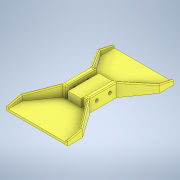
# Autodesk Inventor part: Base
Saved by Autodesk Inventor 2022.4 (Build 264492000, 492)
## iProperties
Created: 2024-03-21
Part Number: Base
Material: Generic
Document SubType Name: Modeling
Designer: t60147996
Density: 1 g/cm^3
Appearance: Smooth - Yellow
Author: t60147996
Autodesk Inventor part; units mm, degrees
ref_plane "YZ Plane" through (0, 0, 0) normal (1, 0, 0) x (0, 1, 0)
ref_plane "XZ Plane" through (0, 0, 0) normal (0, 1, 0) x (-1, 0, 0)
ref_plane "XY Plane" through (0, 0, 0) normal (0, 0, 1) x (1, 0, 0)
sketch "Sketch1" plane through (0, 0, 0) normal (0, 1, 0) x (-1, 0, 0)
  line L0 (88.9, 152.4) -> (-88.9, 152.4)
  line L1 (-88.9, 152.4) -> (-88.9, -152.4)
  line L2 (-88.9, -152.4) -> (88.9, -152.4)
  line L3 (88.9, -152.4) -> (88.9, 152.4)
  line L4 (88.9, 152.4) -> (-88.9, -152.4) construction
  line L5 (-88.9, 152.4) -> (88.9, -152.4) construction
  point P0 (0, 0)
  dimension "d2" = 177.8
  dimension "d3" = 304.8
  constraints: 12 end point, 2 midpoint, 2 parallel, 1 horizontal, 1 perpendicular
  measures "d2" distance of L2.end L1.end
  measures "d3" distance of L1.end L0.end
extrude "Extrusion1" add sketch "Sketch1" along normal blind 38.1
sketch "Sketch2" plane through (0, 38.1, 0) normal (0, 1, 0) x (1, 0, 0)
  line L0 (-88.9, -110.6499) -> (-38.1, -38.1)
  line L1 (-38.1, -38.1) -> (-38.1, 38.1)
  line L2 (-88.9, 152.4) -> (-88.9, -152.4) projected
  line L3 (-38.1, 38.1) -> (-88.9, 110.6499)
  line L4 (-88.9, -110.6499) -> (-88.9, 110.6499)
  point P0 (0, 0)
  point P1 (-38.1, 0)
  point P2 (-88.9, 0)
  point P3 (-88.9, 0)
  dimension "d8" = 50.8
  dimension "d9" = 35
  dimension "d10" = 35
  dimension "d11" = 114.3
  constraints: 8 end point, 3 midpoint, 1 coincident, 1 horizontal alignment, 1 parallel, 1 vertical
  measures "d8" distance between parallel lines of L4 L1
  measures "d9" angle of L4 L3
  measures "d10" angle of L4 L0
  measures "d11" vertical distance of L2.end L0.end
extrude "Extrusion2" cut sketch "Sketch2" against normal blind 38.1
mirror "Mirror1" about plane through (0, 0, 0) normal (1, 0, 0) of "Extrusion2"
sketch "Sketch3" plane through (-88.9, 0, -152.4) normal (-1, 0, 0) x (0, 0, 1)
  line L0 (41.7501, 38.1) -> (114.3, 38.1) projected
  line L1 (114.3, 38.1) -> (0, 12.7)
  line L2 (0, 0) -> (0, 38.1) projected
  line L3 (0, 38.1) -> (41.7501, 38.1) projected
  line L4 (0, 0) -> (41.7501, 0) projected
  point P0 (152.4, 0)
  constraints: 2 end point, 1 point on line
extrude "Extrusion3" cut sketch "Sketch3" against normal through all
mirror "Mirror2" about plane through (0, 0, 0) normal (0, 0, 1) of "Extrusion3"
sketch "Sketch4" plane through (0, 38.1, 0) normal (0, 1, 0) x (1, 0, 0)
  line L0 (88.9, 152.4) -> (88.9, 110.6499) projected
  line L1 (88.9, 110.6499) -> (38.1, 38.1) projected
  line L2 (38.1, 38.1) -> (-38.1, 38.1) projected
  line L3 (-38.1, 38.1) -> (-88.9, 110.6499) projected
  line L4 (-88.9, 110.6499) -> (-88.9, 152.4) projected
  line L5 (-82.55, 175.6071) -> (-82.55, 112.6521)
  line L6 (-82.55, 112.6521) -> (-34.7944, 44.45)
  line L7 (-34.7944, 44.45) -> (34.7944, 44.45)
  line L8 (34.7944, 44.45) -> (82.55, 112.6521)
  line L9 (82.55, 112.6521) -> (82.55, 175.6071)
  line L10 (82.55, 175.6071) -> (-82.55, 175.6071)
  line L11 (-88.9, 152.4) -> (-88.9, 110.6499) projected
  point P0 (0, 0)
  dimension "d18" = 6.35
  constraints: 12 end point, 1 perpendicular, 4 other
  measures "d18" distance between parallel lines of L4 L5
extrude "Extrusion4" cut sketch "Sketch4" against normal blind 31.75
mirror "Mirror3" about plane through (0, 0, 0) normal (0, 0, 1) of "Extrusion4"
sketch "Sketch5" plane through (0, 38.1, 0) normal (0, 1, 0) x (1, 0, 0)
  line L0 (-19.05, 53.7208) -> (-25.4, 53.7208)
  line L1 (-25.4, 53.7208) -> (-25.4, -69.8456)
  line L2 (-25.4, -69.8456) -> (-19.05, -69.8456)
  line L3 (-19.05, -69.8456) -> (-19.05, 53.7208)
  line L4 (-38.1, 38.1) -> (-38.1, -38.1) projected
  point P0 (0, 0)
  dimension "d21" = 6.35
  dimension "d22" = 12.7
  constraints: 8 end point, 2 parallel, 1 horizontal, 1 perpendicular
  measures "d21" distance of L1.end L2.end
  measures "d22" distance between parallel lines of L4 L1
extrude "Extrusion5" cut sketch "Sketch5" against normal blind 31.75
mirror "Mirror4" about plane through (0, 0, 0) normal (1, 0, 0) of "Extrusion5"
sketch "Sketch6" plane through (0, 38.1, 0) normal (0, 1, 0) x (1, 0, 0)
  line L0 (20.5219, 59.3789) -> (-22.204, 59.3789)
  line L1 (-22.204, 59.3789) -> (-22.204, -65.4346)
  line L2 (-22.204, -65.4346) -> (20.5219, -65.4346)
  line L3 (20.5219, -65.4346) -> (20.5219, 59.3789)
  point P0 (0, 0)
  constraints: 8 end point, 2 parallel, 1 horizontal, 1 perpendicular
extrude "Extrusion6" cut sketch "Sketch6" against normal blind 8.89
sketch "Sketch7" plane through (-38.1, 0, -38.1) normal (-1, 0, 0) x (0, 0, 1)
  line L0 (0, 38.1) -> (0, 0) projected
  line L1 (76.2, 38.1) -> (76.2, 0) projected
  line L2 (76.2, 0) -> (0, 0) projected
  point P0 (38.1, 0)
  point P1 (19.05, 21.59)
  point P2 (57.15, 21.59)
  dimension "d27" = 19.05
  dimension "d28" = 19.05
  dimension "d29" = 21.59
  constraints: 1 horizontal alignment
  measures "d27" distance from line of L0 point (19.05, 21.59)
  measures "d28" distance from line of L1 point (57.15, 21.59)
  measures "d29" distance from line of L2 point (19.05, 21.59)
hole "Hole1" at (-38.1, 21.59, -19.05) at (-38.1, 21.59, 19.05) direction (1, 0, 0) diameter 8.89 end through all
fillet "Fillet1" radius 2.54 32 edges at (-58.6722, 29.1109, 78.551) (-63.5, 30.0389, 74.375) (-88.9, 17.3389, 131.525) (-82.55, 17.1164, 132.526) (-85.725, 12.7, 152.4) (58.6722, 29.1109, 78.551) (63.5, 30.0389, 74.375) (82.55, 17.1164, 132.526) (88.9, 17.3389, 131.525) (85.725, 12.7, 152.4) (30.0972, 36.6889, 44.45) (25.4, 38.1, 0) (38.1, 38.1, 0) (30.0972, 36.6889, -44.45) (58.6722, 29.1109, -78.551) (63.5, 30.0389, -74.375) (88.9, 17.3389, -131.525) (85.725, 12.7, -152.4) (82.55, 17.1164, -132.526) (-30.0972, 36.6889, -44.45) (-30.0972, 36.6889, 44.45) (-25.4, 38.1, 0) (-38.1, 38.1, 0) (-58.6722, 29.1109, -78.551) (-63.5, 30.0389, -74.375) (-82.55, 17.1164, -132.526) (-88.9, 17.3389, -131.525) (-85.725, 12.7, -152.4) (-25.4, 37.3944, -41.275) (-25.4, 37.3944, 41.275) (25.4, 37.3944, 41.275) (25.4, 37.3944, -41.275)
body "Solid1"
